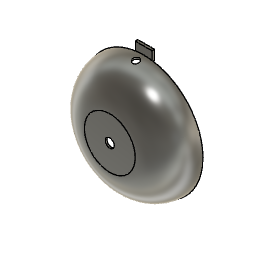
dumb_doorbell (Autodesk Fusion 360 design; units mm, degrees)
Autodesk Fusion 360 part; units mm, degrees
sketch "Sketch1" plane through (0, 0, 0) normal (0, 0, 1) x (1, 0, 0)
  line L0 (0, 0) -> (15.001, 0)
  line L1 (35, 19.999) -> (35, 20)
  arc A0 (15.001, 0) -> (35, 19.999) centre (15.001, 19.999) ccw
  line L2 (0, 1) -> (15.001, 1)
  arc A1 (15.001, 1) -> (34, 19.999) centre (15.001, 19.999) ccw
  line L3 (34, 19.999) -> (34, 20)
  line L4 (34, 20) -> (35, 20)
  line L5 (0, 1) -> (0, 0)
  point P0 (35, 0)
  dimension "d1" = 35
  dimension "d2" = 20
  dimension "d3" = 19.999
  dimension "d4" = -1
  constraint horizontal L0
  constraint vertical L1
  constraint coincident L0.start L5.end
  constraint coincident P0 L1
  constraint coincident P0 L0
  constraint tangent L1 A0
  constraint tangent L0 A0
  constraint perpendicular L1 L4
  constraint perpendicular L0 L5
  measures "d1" distance of L0.start P0
  measures "d2" distance of P0 L1.end
  measures "d3" radius of A0
revolve "Revolve1" add sketch "Sketch1" angle 360 about axis through (0, 1.75, 0) along (0, 1, 0)
ref_plane "WorkPlane1" through (0, 0, 35) normal (0, 0, 1) x (1, 0, 0)
sketch "Sketch2" plane through (0, 0, 35) normal (0, 0, 1) x (1, 0, 0)
  line L0 (0, 0) -> (0, 15.5)
  circle A0 centre (0, 15.5) radius 1.95
  dimension "d7" = 15.5
  dimension "d8" = 3.9
  constraint coincident L0.start origin
  constraint vertical L0
  constraint coincident L0.end A0.centre
  measures "d7" distance of L0.start L0.end
  measures "d8" diameter of A0
extrude "Extrude1" cut sketch "Sketch2" against normal blind 10
sketch "Sketch3" plane through (0, 0, 0) normal (0, -1, 0) x (1, 0, 0)
  circle A0 centre (0, 0) radius 15.001
  circle A1 centre (0, 0) radius 2.65
  dimension "d11" = 5.3
  constraint coincident A0.centre A1.centre
  measures "d11" diameter of A1
extrude "Extrude2" cut sketch "Sketch3" along normal blind 30 and the other way blind 30 contours A1
sketch "Sketch4" plane through (0, 20, 0) normal (0, 1, 0) x (-1, 0, 0)
  circle A0 centre (0, 0) radius 34
  circle A1 centre (0, 0) radius 35
  line L0 (-5, 39.6303) -> (5, 39.6303)
  line L1 (5, 39.6303) -> (5, 33.6303)
  line L2 (-5, 33.6303) -> (-5, 39.6303)
  line L3 (-5, 39.6303) -> (0, 34) construction
  line L4 (5, 39.6303) -> (0, 34) construction
  line L5 (0, 34) -> (-5, 34)
  line L6 (0, 34) -> (5, 34)
  dimension "d16" = 6
  constraint horizontal L0
  constraint perpendicular L0 L1
  constraint parallel L1 L2
  constraint coincident A0 L3.end
  constraint coincident L3.end L4.end
  constraint coincident A0 L1.end
  constraint coincident L1 L6.end
  constraint coincident A0 L2.start
  constraint coincident L2 L5.end
  measures "d16" distance of L0.start L2.start
extrude "Extrude3" add sketch "Sketch4" along normal blind 1.5 contours A1 L1 L2 L5 L6 | A1 L0 L1 L2
